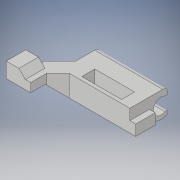
# Autodesk Inventor part: 30_Switch
Saved by Autodesk Inventor 2019 (Build 230136000, 136)
## iProperties
Created: 2019-10-09
Part Number: 30_Switch
Material: Generic
Document SubType Name: Modeling
Designer: James
Density: 1 g/cm^3
Appearance: Default
Author: James
Autodesk Inventor part; units mm, degrees
ref_plane "YZ Plane" through (0, 0, 0) normal (1, 0, 0) x (0, 1, 0)
ref_plane "XZ Plane" through (0, 0, 0) normal (0, 1, 0) x (-1, 0, 0)
ref_plane "XY Plane" through (0, 0, 0) normal (0, 0, 1) x (1, 0, 0)
sketch "Sketch1" plane through (0, 0, 0) normal (1, 0, 0) x (0, 1, 0)
  arc A0 (3.4641, -2) -> (-3.4641, -2) centre (0, 0) ccw
  arc A1 (3.4641, -2) -> (5.1962, -3) centre (4.3301, -2.5) ccw
  arc A2 (-5.1962, -3) -> (-3.4641, -2) centre (-4.3301, -2.5) ccw
  line L0 (7, 16) -> (-4, 16)
  line L1 (-4, 16) -> (-4, 4.4721)
  line L2 (4.4721, 4) -> (7, 4)
  line L3 (7, 4) -> (7, 16)
  arc A3 (5.1962, -3) -> (5.8413, 1.3709) centre (0, 0) ccw
  arc A4 (-4, 4.4721) -> (-5.1962, -3) centre (0, 0) ccw
  line L4 (7, 4) -> (7, -0.8301)
  arc A5 (4.3301, -3.5) -> (7, -0.8301) centre (4.3301, -0.8301) ccw
  dimension "d0" = 8
  dimension "d4" = 2.5
  dimension "d5" = 7
  dimension "d6" = 12
  dimension "d7" = 11
  dimension "d34" = 6
  dimension "d35" = 6
  constraints: 14 point on circle, 10 end point, 7 tangent, 6 centre point, 2 coincident, 2 parallel, 1 horizontal, 1 horizontal alignment, 1 perpendicular, 1 vertical, 1 vertical alignment
  measures "d0" diameter of A0
  measures "d4" vertical distance of A1.centre point (0, 0)
  measures "d5" distance from line of point (0, 0) L3
  measures "d6" distance of L2.end L0.start
  measures "d7" distance of L0.start L0.end
  measures "d34" radius of A3
  measures "d35" radius of A4
extrude "Extrusion1" add sketch "Sketch1" along normal blind 38.8
fillet "Fillet1" radius 2 1 edges at (19.4, -4, 4.4721)
sketch "Sketch2" plane through (38.8, 0, 0) normal (1, 0, 0) x (0, 0, -1)
  line L0 (-16, -4) -> (-5.2915, -4) projected
  line L1 (-16, -4) -> (-6, -4)
  line L2 (-6, -4) -> (-6, 1.5)
  line L3 (-6, 1.5) -> (-16, 1.5)
  line L4 (-16, 1.5) -> (-16, -4)
  point P0 (0, 0)
  dimension "d11" = 10
  dimension "d12" = 5.5
  constraints: 8 end point, 2 parallel, 1 horizontal, 1 perpendicular
  measures "d11" distance of L2.end L3.end
  measures "d12" distance of L3.end L0.start
extrude "Extrusion2" add sketch "Sketch2" along normal blind 3
sketch "Sketch3" plane through (0, 0, 0) normal (-1, 0, 0) x (0, 0, 1)
  point P0 (0, 0)
sketch "Sketch4" plane through (0, 0, 0) normal (-1, 0, 0) x (0, 0, 1)
  line L0 (16, -4) -> (6, -4)
  line L1 (6, -4) -> (6, 7)
  line L2 (6, 7) -> (16, 7)
  line L3 (16, 7) -> (16, -4)
  point P0 (0, 0)
  dimension "d15" = 10
  dimension "d16" = 11
  constraints: 8 end point, 2 parallel, 2 point on line, 1 horizontal, 1 perpendicular
  measures "d15" distance of L1.end L2.end
  measures "d16" distance of L2.end L0.start
extrude "Extrusion3" add sketch "Sketch4" along normal blind 4
sketch "Sketch8" plane through (-4, 0, 0) normal (-1, 0, 0) x (0, 0, 1)
  line L0 (20, 10.3) -> (30, 10.3)
  line L1 (30, 10.3) -> (30, 2.5)
  line L2 (30, 2.5) -> (20, 2.5)
  line L3 (20, 2.5) -> (20, 10.3)
  point P0 (0, 0)
  dimension "d26" = 7.8
  dimension "d27" = 10.3
  dimension "d28" = 20
  dimension "d29" = 10
  constraints: 8 end point, 2 parallel, 1 horizontal, 1 perpendicular
  measures "d26" distance of L0.end L1.end
  measures "d27" distance from line of point (0, 0) L0
  measures "d28" distance from line of L3 point (0, 0)
  measures "d29" distance of L0.start L0.end
extrude "Extrusion6" add sketch "Sketch8" along normal blind 6.5
sketch "Sketch9" plane through (-4, 0, 0) normal (1, 0, 0) x (0, 0, -1)
  line L0 (-30, 2.5) -> (-20, 2.5) projected
  line L1 (-16, 7) -> (-16, 1.5) projected
  line L2 (-30, 2.5) -> (-16, 2.5)
  line L3 (-16, 2.5) -> (-16, 7)
  line L4 (-16, 7) -> (-30, 7)
  line L5 (-30, 7) -> (-30, 2.5)
  point P0 (0, 0)
  constraints: 8 end point, 2 parallel, 1 horizontal, 1 perpendicular
extrude "Extrusion7" add sketch "Sketch9" along normal blind 6
sketch "Sketch11" plane through (0, 7, 6) normal (0, 1, 0) x (1, 0, 0)
  line L0 (32.8, -8.2459) -> (12.4, -8.2459)
  line L1 (12.4, -8.2459) -> (12.4, -1.5459)
  line L2 (12.4, -1.5459) -> (32.8, -1.5459)
  line L3 (32.8, -1.5459) -> (32.8, -8.2459)
  line L4 (38.8, 6.8301) -> (38.8, -10) projected
  point P0 (0, 6)
  point P1 (38.8, 2)
  dimension "d47" = 20.4
  dimension "d48" = 6.7
  dimension "d67" = 6
  constraints: 8 end point, 2 parallel, 1 horizontal, 1 perpendicular
  measures "d47" distance of L0.start L0.end
  measures "d48" distance of L0.end L1.end
  measures "d67" distance between parallel lines of L4 L3
extrude "Extrusion9" cut sketch "Sketch11" against normal blind 10
sketch "Sketch12" plane through (0, -3, 6) normal (0, 1, 0) x (1, 0, 0)
  line L0 (11.9901, -47.107) -> (11.9901, -26.707)
  line L1 (18.6901, -26.707) -> (18.6901, -47.107)
  line L2 (11.9901, -46.407) -> (18.6901, -46.407)
  line L3 (18.6901, -46.407) -> (18.6901, -43.207)
  line L4 (18.6901, -43.207) -> (11.9901, -43.207)
  line L5 (11.9901, -43.207) -> (11.9901, -46.407)
  line L6 (11.9901, -39.107) -> (18.6901, -39.107)
  line L7 (18.6901, -39.107) -> (18.6901, -35.907)
  line L8 (18.6901, -35.907) -> (11.9901, -35.907)
  line L9 (11.9901, -35.907) -> (11.9901, -39.107)
  line L10 (11.9901, -30.307) -> (18.6901, -30.307)
  line L11 (18.6901, -30.307) -> (18.6901, -27.107)
  line L12 (18.6901, -27.107) -> (11.9901, -27.107)
  line L13 (11.9901, -27.107) -> (11.9901, -30.307)
  line L14 (18.6901, -47.107) -> (11.9901, -47.107)
  line L15 (11.9901, -26.707) -> (18.6901, -26.707)
  line L16 (32.8, -8.2459) -> (12.4, -8.2459) projected
  line L17 (12.4, -1.5459) -> (32.8, -1.5459) projected
  line L18 (12.8, -8.2459) -> (16, -8.2459)
  line L19 (16, -8.2459) -> (16, -1.5459)
  line L20 (16, -1.5459) -> (12.8, -1.5459)
  line L21 (12.8, -1.5459) -> (12.8, -8.2459)
  line L22 (21.6, -8.2459) -> (24.8, -8.2459)
  line L23 (24.8, -8.2459) -> (24.8, -1.5459)
  line L24 (24.8, -1.5459) -> (21.6, -1.5459)
  line L25 (21.6, -1.5459) -> (21.6, -8.2459)
  line L26 (32.1, -8.2459) -> (28.9, -8.2459)
  line L27 (28.9, -8.2459) -> (28.9, -1.5459)
  line L28 (28.9, -1.5459) -> (32.1, -1.5459)
  line L29 (32.1, -1.5459) -> (32.1, -8.2459)
  line L30 (12.4, -8.2459) -> (12.4, -1.5459) projected
  point P0 (0, 6)
  point P1 (15.3401, -24.907)
  point P2 (11.9901, -44.807)
  point P3 (11.9901, -37.507)
  point P4 (11.9901, -28.707)
  point P5 (14.4, -8.2459)
  point P6 (23.2, -8.2459)
  point P7 (30.5, -8.2459)
  dimension "d51" = 7.3
  dimension "d52" = 8.8
  dimension "d53" = 3.2
  dimension "d54" = 3.2
  dimension "d55" = 3.2
  dimension "d56" = 2
  dimension "d59" = 3.2
  dimension "d60" = 3.2
  dimension "d61" = 3.2
  dimension "d62" = 8.8
  dimension "d63" = 7.3
  dimension "d64" = 2
  constraints: 56 end point, 12 parallel, 12 point on line, 6 horizontal, 6 midpoint, 6 perpendicular
  measures "d51" distance of point (11.99, -37.507) point (11.99, -44.807)
  measures "d52" distance of point (11.99, -28.707) point (11.99, -37.507)
  measures "d53" distance between parallel lines of L4 L2
  measures "d54" distance of L8.end L6.start
  measures "d55" distance between parallel lines of L10 L12
  measures "d56" distance from line of L15 point (11.99, -28.707)
  measures "d59" distance of L18.start L18.end
  measures "d60" distance between parallel lines of L23 L25
  measures "d61" distance between parallel lines of L29 L27
  measures "d62" distance of point (23.2, -8.246) point (14.4, -8.246)
  measures "d63" distance of point (30.5, -8.246) point (23.2, -8.246)
  measures "d64" distance from line of L30 point (14.4, -8.246)
extrude "Extrusion10" cut sketch "Sketch12" against normal blind 10 contours L16 L27 L17 L29 | L16 L25 L17 L23 | L16 L21 L17 L19
sketch "Sketch13" plane through (0, 0, 0) normal (-1, 0, 0) x (0, 0, 1)
  line L0 (-8.6099, 16.8376) -> (10, 16.8376)
  line L1 (10, -12.4202) -> (-8.6099, -12.4202)
  line L2 (-8.6099, -12.4202) -> (-8.6099, 16.8376)
  line L3 (10, 16.8376) -> (10, -12.4202)
  line L4 (16, -4) -> (16, 2.5) projected
  point P0 (0, 0)
  point P1 (16, 0.5)
  dimension "d70" = 6
  constraints: 8 end point, 1 horizontal, 1 parallel, 1 perpendicular
  measures "d70" distance between parallel lines of L3 L4
extrude "Extrusion11" cut sketch "Sketch13" along normal mid plane 8
chamfer "Chamfer1" distance 4 angle 45 2 edges at (4, 1.5, 10) (-4, 1.5, 10)
chamfer "Chamfer2" distance 5.75 angle 45 1 edges at (2, 4.75, 16)
chamfer "Chamfer3" distance 3.3 angle 45 1 edges at (-4, 7, 25)
chamfer "Chamfer4" distance 6.5 angle 45 2 edges at (4.875, 2.5, 16) (-1, 2.5, 16)
sketch "Sketch14" plane through (38.8, 7, 16) normal (0, 1, 0) x (1, 0, 0)
  line L0 (-34.8, 10) -> (-34.8, 10.7085) projected
  line L1 (-34.8, 10) -> (-34.8, 7)
  line L2 (-34.8, 7) -> (-42.8, -1)
  line L3 (-42.8, 2) -> (-42.8, -4) projected
  line L4 (-42.8, 2) -> (-34.8, 10) projected
  line L5 (-42.8, 2) -> (-42.8, -1)
  line L6 (-42.8, 2) -> (-34.8, 10)
  line L7 (-42.8, -4) -> (-49.3, -4) projected
  point P0 (-38.8, 16)
  dimension "d85" = 3
  constraints: 8 end point, 3 equal length, 1 midpoint, 1 vertical
  measures "d85" distance from line of L7 L2.end
extrude "Extrusion12" cut sketch "Sketch14" against normal blind 15
sketch "Sketch15" plane through (-10.5, 2.5, 30) normal (0, 0, 1) x (1, 0, 0)
  line L0 (0, 0) -> (12.5, 0) projected
  line L1 (6.5, -2.5) -> (6.5, -5.5) projected
  line L2 (0, 0) -> (6.5, 0)
  line L3 (6.5, 0) -> (6.5, -5.5)
  line L4 (6.5, -5.5) -> (0, -5.5)
  line L5 (0, -5.5) -> (0, 0)
  point P0 (10.5, -2.5)
  constraints: 8 end point, 2 parallel, 1 horizontal, 1 perpendicular
extrude "Extrusion13" cut sketch "Sketch15" against normal blind 30.25
body "Solid1"
